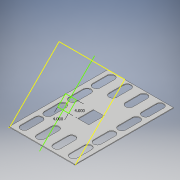
# Autodesk Inventor part: Top
Saved by Autodesk Inventor 2019 (Build 230136000, 136)
## iProperties
Created: 2021-09-15
Part Number: Top
Material: Generic
Document SubType Name: Modeling
Designer: timmy
Density: 1 g/cm^3
Appearance: Default
Author: timmy
Autodesk Inventor part; units mm, degrees
ref_plane "YZ Plane" through (0, 0, 0) normal (1, 0, 0) x (0, 1, 0)
ref_plane "XZ Plane" through (0, 0, 0) normal (0, 1, 0) x (-1, 0, 0)
ref_plane "XY Plane" through (0, 0, 0) normal (0, 0, 1) x (1, 0, 0)
sketch "Sketch1" plane through (0, 0, 0) normal (0, 1, 0) x (-1, 0, 0)
  line L0 (0, 0) -> (-609.6, 0)
  line L1 (-609.6, 0) -> (-609.6, -914.4)
  line L2 (-609.6, -914.4) -> (0, -914.4)
  line L3 (0, -914.4) -> (0, 0)
  dimension "d0" = 609.6
  dimension "d1" = 914.4
  constraints: 8 end point, 2 parallel, 1 horizontal, 1 perpendicular
  measures "d0" distance of L2.end L1.end
  measures "d1" distance of L1.end L0.end
extrude "Extrusion1" add sketch "Sketch1" along normal blind 6.35
ref_plane "Work Plane1" through (0, 0, 0) normal (0, 0.7071068, 0.7071068) x (1, 0, 0)
sketch "Sketch3" plane through (0, 0, 0) normal (0, 0.7071068, 0.7071068) x (1, 0, 0)
  line L0 (0, 4.4901) -> (609.6, 4.4901) projected
  line L1 (609.6, 4.4901) -> (609.6, 651.0686) projected
  line L2 (609.6, 651.0686) -> (0, 651.0686) projected
  line L3 (0, 651.0686) -> (0, 4.4901) projected
  line L4 (0, 4.4901) -> (609.6, 4.4901) projected
  line L5 (304.8, -36.3031) -> (304.8, 687.2508)
  line L6 (254, 376.2738) -> (355.6, 376.2738)
  line L7 (355.6, 376.2738) -> (355.6, 274.6738)
  line L8 (355.6, 274.6738) -> (254, 274.6738)
  line L9 (254, 274.6738) -> (254, 376.2738)
  line L10 (254, 376.2738) -> (355.6, 274.6738) construction
  line L11 (355.6, 376.2738) -> (254, 274.6738) construction
  point P0 (0, 0)
  point P1 (304.8, 325.4738)
  dimension "d5" = 101.6
  dimension "d6" = 101.6
  constraints: 14 end point, 3 midpoint, 2 parallel, 1 horizontal, 1 perpendicular, 1 vertical
  measures "d5" distance of L7.end L8.end
  measures "d6" distance of L6.end L7.end
extrude "Extrusion2" cut sketch "Sketch3" against normal up to surface contours L8 L9 L6 L5 | L5 L6 L7 L8 surface through (304.8, 0, -457.2) normal (0, 1, 0)
sketch "Sketch4" plane through (0, 6.35, 0) normal (0, 1, 0) x (1, 0, 0)
  line L0 (111.5231, 866.3769) -> (111.5231, 733.8231)
  arc A0 (40.8769, 733.8231) -> (111.5231, 733.8231) centre (76.2, 733.8231) ccw
  line L1 (40.8769, 733.8231) -> (40.8769, 866.3769)
  arc A1 (111.5231, 866.3769) -> (40.8769, 866.3769) centre (76.2, 866.3769) ccw
  line L2 (0, 0) -> (609.6, 0) construction
  line L3 (193.2769, 866.3769) -> (193.2769, 733.8231)
  arc A2 (193.2769, 733.8231) -> (263.9231, 733.8231) centre (228.6, 733.8231) ccw
  line L4 (263.9231, 733.8231) -> (263.9231, 866.3769)
  arc A3 (263.9231, 866.3769) -> (193.2769, 866.3769) centre (228.6, 866.3769) ccw
  line L5 (111.5231, 513.0358) -> (111.5231, 645.5897)
  arc A4 (111.5231, 645.5897) -> (40.8769, 645.5897) centre (76.2, 645.5897) ccw
  line L6 (40.8769, 645.5897) -> (40.8769, 513.0358)
  arc A5 (40.8769, 513.0358) -> (111.5231, 513.0358) centre (76.2, 513.0358) ccw
  line L7 (498.0769, 866.3769) -> (498.0769, 733.8231)
  arc A6 (498.0769, 733.8231) -> (568.7231, 733.8231) centre (533.4, 733.8231) ccw
  line L8 (568.7231, 733.8231) -> (568.7231, 866.3769)
  arc A7 (568.7231, 866.3769) -> (498.0769, 866.3769) centre (533.4, 866.3769) ccw
  line L9 (416.3231, 866.3769) -> (416.3231, 733.8231)
  arc A8 (345.6769, 733.8231) -> (416.3231, 733.8231) centre (381, 733.8231) ccw
  line L10 (345.6769, 733.8231) -> (345.6769, 866.3769)
  arc A9 (416.3231, 866.3769) -> (345.6769, 866.3769) centre (381, 866.3769) ccw
  line L11 (498.0769, 513.0358) -> (498.0769, 645.5897)
  arc A10 (568.7231, 645.5897) -> (498.0769, 645.5897) centre (533.4, 645.5897) ccw
  line L12 (568.7231, 645.5897) -> (568.7231, 513.0358)
  arc A11 (498.0769, 513.0358) -> (568.7231, 513.0358) centre (533.4, 513.0358) ccw
  line L13 (111.5231, 63.6485) -> (111.5231, 196.2024)
  arc A12 (111.5231, 196.2024) -> (40.8769, 196.2024) centre (76.2, 196.2024) ccw
  line L14 (40.8769, 196.2024) -> (40.8769, 63.6485)
  arc A13 (40.8769, 63.6485) -> (111.5231, 63.6485) centre (76.2, 63.6485) ccw
  line L15 (193.2769, 63.6485) -> (193.2769, 196.2024)
  arc A14 (263.9231, 196.2024) -> (193.2769, 196.2024) centre (228.6, 196.2024) ccw
  line L16 (263.9231, 196.2024) -> (263.9231, 63.6485)
  arc A15 (193.2769, 63.6485) -> (263.9231, 63.6485) centre (228.6, 63.6485) ccw
  line L17 (111.5231, 416.9897) -> (111.5231, 284.4358)
  arc A16 (40.8769, 284.4358) -> (111.5231, 284.4358) centre (76.2, 284.4358) ccw
  line L18 (40.8769, 284.4358) -> (40.8769, 416.9897)
  arc A17 (111.5231, 416.9897) -> (40.8769, 416.9897) centre (76.2, 416.9897) ccw
  line L19 (498.0769, 63.6485) -> (498.0769, 196.2024)
  arc A18 (568.7231, 196.2024) -> (498.0769, 196.2024) centre (533.4, 196.2024) ccw
  arc A19 (498.0769, 284.4358) -> (568.7231, 284.4358) centre (533.4, 284.4358) ccw
  line L20 (568.7231, 196.2024) -> (568.7231, 63.6485)
  arc A20 (498.0769, 63.6485) -> (568.7231, 63.6485) centre (533.4, 63.6485) ccw
  arc A21 (416.3231, 196.2024) -> (345.6769, 196.2024) centre (381, 196.2024) ccw
  line L21 (416.3231, 63.6485) -> (416.3231, 196.2024)
  line L22 (345.6769, 196.2024) -> (345.6769, 63.6485)
  arc A22 (345.6769, 63.6485) -> (416.3231, 63.6485) centre (381, 63.6485) ccw
  line L23 (498.0769, 416.9897) -> (498.0769, 284.4358)
  line L24 (568.7231, 284.4358) -> (568.7231, 416.9897)
  arc A23 (568.7231, 416.9897) -> (498.0769, 416.9897) centre (533.4, 416.9897) ccw
  point P0 (0, 914.4)
  constraints: 48 end point, 48 point on circle, 24 centre point
extrude "Extrusion3" cut sketch "Sketch4" against normal blind 6.35
body "Solid1"
